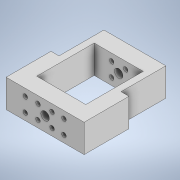
# Autodesk Inventor part: 20220612_サーボ仮
Saved by Autodesk Inventor 2020 (Build 240168000, 168)
## iProperties
Created: 2022-06-10
Part Number: 20220612_サーボ仮
Material: 一般
Document SubType Name: Modeling
Designer: Naggy
Density: 1 g/cm^3
Appearance: 既定
Author: Naggy
Autodesk Inventor part; units mm, degrees
ref_plane "YZ Plane" through (0, 0, 0) normal (1, 0, 0) x (0, 1, 0)
ref_plane "XZ Plane" through (0, 0, 0) normal (0, 1, 0) x (-1, 0, 0)
ref_plane "XY Plane" through (0, 0, 0) normal (0, 0, 1) x (1, 0, 0)
sketch "スケッチ1" plane through (0, 0, 0) normal (0, 0, 1) x (1, 0, 0)
  line L0 (-22.1, -10) -> (22.1, -10)
  line L1 (22.1, -10) -> (22.1, 10)
  line L2 (22.1, 10) -> (-22.1, 10)
  line L3 (-22.1, 10) -> (-22.1, -10)
  line L4 (-22.1, -10) -> (22.1, 10) construction
  line L5 (22.1, -10) -> (-22.1, 10) construction
  point P0 (0, 0)
  dimension "d0" = 44.2
  dimension "d1" = 20
  constraints: 12 end point, 2 midpoint, 2 parallel, 1 horizontal, 1 perpendicular
  measures "d0" distance between parallel lines of L1 L3
  measures "d1" distance between parallel lines of L0 L2
extrude "押し出し1" add sketch "スケッチ1" along normal blind 32
sketch "スケッチ2" plane through (0, 0, 32) normal (0, 0, 1) x (1, 0, 0)
  line L0 (-27.8, -10) -> (27.8, -10)
  line L1 (27.8, -10) -> (27.8, 10)
  line L2 (27.8, 10) -> (-27.8, 10)
  line L3 (-27.8, 10) -> (-27.8, -10)
  line L4 (-27.8, -10) -> (27.8, 10) construction
  line L5 (27.8, -10) -> (-27.8, 10) construction
  point P0 (0, 0)
  dimension "d4" = 20
  dimension "d5" = 55.6
  constraints: 12 end point, 2 midpoint, 2 parallel, 1 horizontal, 1 perpendicular
  measures "d4" distance between parallel lines of L0 L2
  measures "d5" distance between parallel lines of L3 L1
extrude "押し出し2" add sketch "スケッチ2" along normal blind 32
sketch "スケッチ3" plane through (0, 0, 0) normal (0, 1, 0) x (-1, 0, 0)
  line L0 (22.1, 0) -> (22.1, 32) projected
  line L1 (-17.5, 7.4854) -> (17.5, 7.4854)
  line L2 (17.5, 7.4854) -> (17.5, 56.5146)
  line L3 (17.5, 56.5146) -> (-17.5, 56.5146)
  line L4 (-17.5, 56.5146) -> (-17.5, 7.4854)
  line L5 (-17.5, 7.4854) -> (17.5, 56.5146) construction
  line L6 (17.5, 7.4854) -> (-17.5, 56.5146) construction
  line L7 (-17.5, 11.5146) -> (17.5, 11.5146)
  line L8 (17.5, 11.5146) -> (17.5, 52.4854)
  line L9 (17.5, 52.4854) -> (-17.5, 52.4854)
  line L10 (-17.5, 52.4854) -> (-17.5, 11.5146)
  line L11 (-17.5, 11.5146) -> (17.5, 52.4854) construction
  line L12 (17.5, 11.5146) -> (-17.5, 52.4854) construction
  point P0 (0, 0)
  point P1 (0, 32)
  dimension "d8" = 22.1
  dimension "d9" = 32
  dimension "d10" = 35
  dimension "d11" = 45
  constraints: 24 end point, 4 midpoint, 4 parallel, 2 horizontal, 2 perpendicular, 1 point on line
  measures "d8" distance from line of point (0, 32) L0
  measures "d9" distance of point (0, 0) point (0, 32)
  measures "d10" distance between parallel lines of L4 L2
  measures "d11" distance between parallel lines of L1 L9
extrude "押し出し3" cut sketch "スケッチ3" against normal mid plane 32 contours L4 L9 L2 L7
sketch "スケッチ4" plane through (0, 0, 0) normal (0, 0, -1) x (-1, 0, 0)
  point P0 (0, 0)
  point P1 (0, 0)
  constraints: 1 coincident
hole "穴1" at (0, 0, 0) direction (0, 0, 1) diameter 6 depth 15 tip angle 118
sketch "スケッチ5" plane through (0, 0, 0) normal (0, 0, -1) x (-1, 0, 0)
  point P0 (0, 0)
  point P1 (-5, 5)
  point P2 (-5, -5)
  point P3 (5.0409, -5)
  point P4 (5, 5)
  dimension "d21" = 5
  dimension "d22" = 5
  dimension "d23" = 5
  dimension "d24" = 5
  dimension "d25" = 5.0409
  dimension "d26" = 5
  measures "d21" horizontal distance of point (-5, 5) point (0, 0)
  measures "d22" horizontal distance of point (-5, 5) point (0, 0)
  measures "d23" horizontal distance of point (-5, -5) point (0, 0)
  measures "d24" horizontal distance of point (-5, -5) point (0, 0)
  measures "d25" horizontal distance of point (5.041, -5) point (0, 0)
  measures "d26" horizontal distance of point (5, 5) point (0, 0)
hole "穴2" at (5, 5, 0) at (5, -5, 0) at (-5.0409, -5, 0) at (-5, 5, 0) direction (0, 0, 1) diameter 3.2 depth 15 tip angle 118
sketch "スケッチ6" plane through (0, 0, 64) normal (0, 0, 1) x (1, 0, 0)
  point P0 (0, 0)
  point P1 (0, 0)
  constraints: 1 coincident
hole "穴3" at (0, 0, 64) direction (0, 0, -1) diameter 6 depth 15 tip angle 118
sketch "スケッチ7" plane through (0, 0, 64) normal (0, 0, 1) x (1, 0, 0)
  circle A0 centre (-5.0409, -5) radius 1.6 projected
  circle A1 centre (-5, 5) radius 1.6 projected
  circle A2 centre (5, 5) radius 1.6 projected
  circle A3 centre (5, -5) radius 1.6 projected
  point P0 (0, 0)
  point P1 (-14.0582, -5)
  point P2 (-14.0582, 5)
  point P3 (13.4789, 5)
  point P4 (13.4789, -5)
  constraints: 4 coincident
hole "穴4" at (-5.0409, -5, 64) at (-5, 5, 64) at (5, 5, 64) at (5, -5, 64) at (-14.0582, -5, 64) at (-14.0582, 5, 64) at (13.4789, 5, 64) at (13.4789, -5, 64) direction (0, 0, -1) diameter 3.2 depth 17.1 tip angle 118
